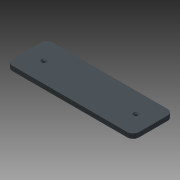
# Autodesk Inventor part: 13_1087_038
Saved by Autodesk Inventor 2014 (Build 180170000, 170)
## iProperties
Created: 2013-09-20
Part Number: 13_1087_038
Material: Allgemein
Document SubType Name: Modeling
Designer: vogel
Density: 1 g/cm^3
Appearance: Eisen - grau
Author: vogel
Autodesk Inventor part; units mm, degrees
ref_plane "YZ Plane" through (0, 0, 0) normal (1, 0, 0) x (0, 1, 0)
ref_plane "XZ Plane" through (0, 0, 0) normal (0, 1, 0) x (-1, 0, 0)
ref_plane "XY Plane" through (0, 0, 0) normal (0, 0, 1) x (1, 0, 0)
sketch "Skizze1" plane through (0, 0, 0) normal (0, 0, 1) x (1, 0, 0)
  line L0 (-78.4497, 0) -> (78.4497, 0) projected
  line L1 (0, -25.9497) -> (0, 25.9497) projected
  line L2 (-50, 17.5) -> (50, 17.5)
  line L3 (55, 12.5) -> (55, -12.5)
  line L4 (50, -17.5) -> (-50, -17.5)
  line L5 (-55, -12.5) -> (-55, 12.5)
  arc A0 (-50, 17.5) -> (-55, 12.5) centre (-50, 12.5) ccw
  arc A1 (-55, -12.5) -> (-50, -17.5) centre (-50, -12.5) ccw
  arc A2 (50, -17.5) -> (55, -12.5) centre (50, -12.5) ccw
  arc A3 (55, 12.5) -> (50, 17.5) centre (50, 12.5) ccw
  point P0 (0, 0)
  point P1 (-55, 17.5)
  point P2 (55, 17.5)
  point P3 (-55, -17.5)
  dimension "d0" = 110
  dimension "d1" = 35
  dimension "d2" = 5
  constraints: 8 end point, 8 point on circle, 8 tangent, 6 point on line, 4 centre point, 3 equal radius, 2 parallel, 1 horizontal, 1 perpendicular, 2 other
  measures "d0" distance of point (-55, 17.5) point (55, 17.5)
  measures "d1" distance of point (-55, -17.5) point (-55, 17.5)
  measures "d2" radius of A0
extrude "Extrusion1" add sketch "Skizze1" along normal blind 4
sketch "Skizze2" plane through (0, 0, 4) normal (0, 0, 1) x (1, 0, 0)
  line L0 (-55, 12.5) -> (-55, -12.5) projected
  line L1 (55, -12.5) -> (55, 12.5) projected
  line L2 (-55, 0) -> (55, 0)
  line L3 (-77, 0) -> (77, 0) projected
  line L4 (0, -24.5) -> (0, 24.5) projected
  point P0 (0, 0)
  point P1 (-40, 0)
  point P2 (40, 0)
  dimension "d5" = 80
  constraints: 2 end point, 2 midpoint, 2 point on line, 1 symmetric about line
  measures "d5" distance of point (40, 0) point (-40, 0)
hole "Bohrung1" at (-40, 0, 4) at (40, 0, 4) direction (0, 0, -1) diameter 2.4 end through all countersink diameter 4.5 countersink angle 90
